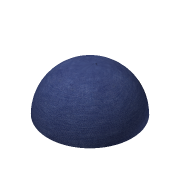
# Autodesk Inventor part: Umbrella
Saved by Autodesk Inventor 2015 (Build 190159000, 159)
## iProperties
Created: 2015-01-31
Part Number: Umbrella
Material: Generic
Document SubType Name: Modeling
Designer: Tanner
Density: 1 g/cm^3
Appearance: Denim - Blue
Author: Tanner
Autodesk Inventor part; units mm, degrees
ref_plane "YZ Plane" through (0, 0, 0) normal (1, 0, 0) x (0, 1, 0)
ref_plane "XZ Plane" through (0, 0, 0) normal (0, 1, 0) x (-1, 0, 0)
ref_plane "XY Plane" through (0, 0, 0) normal (0, 0, 1) x (1, 0, 0)
sketch "Sketch1" plane through (0, 0, 0) normal (0, 0, 1) x (1, 0, 0)
  line L0 (0, 0) -> (-127, 0)
  line L1 (0, 0) -> (0, 127)
  arc A0 (0, 127) -> (-127, 0) centre (0, 0) ccw
  dimension "d0" = 127
  dimension "d1" = 127
  dimension "d2" = 90
  dimension "d3" = 127
  constraints: 4 end point, 2 point on circle, 1 centre point, 1 horizontal
  measures "d0" distance of L0.start L0.end
  measures "d1" distance of L0.start L1.end
  measures "d2" angle of L0 L1
  measures "d3" radius of A0
revolve "Revolution1" add sketch "Sketch1" angle 360 about axis through (0, 0, 0) along (0, 1, 0)
body "Solid1"
